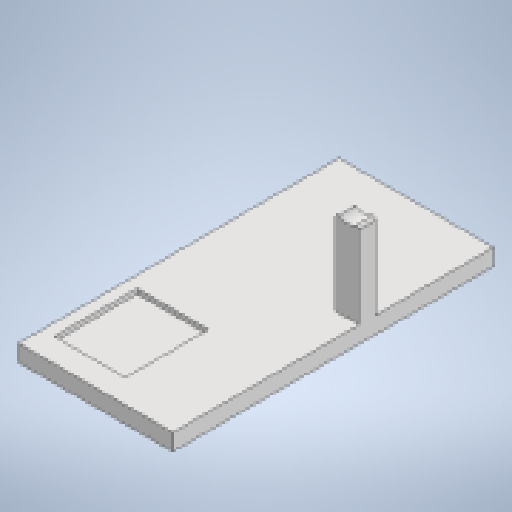
# Autodesk Inventor part: body-1
Saved by Autodesk Inventor 2025 (Build 290162000, 162)
## iProperties
Created: 2026-01-27
Part Number: body-1
Material: 一般
Document SubType Name: Modeling
Designer: mahhy
Density: 1 g/cm^3
Appearance: 既定
Author: mahhy
Autodesk Inventor part; units mm, degrees
ref_plane "YZ Plane" through (0, 0, 0) normal (1, 0, 0) x (0, 1, 0)
ref_plane "XZ Plane" through (0, 0, 0) normal (0, 1, 0) x (-1, 0, 0)
ref_plane "XY Plane" through (0, 0, 0) normal (0, 0, 1) x (1, 0, 0)
sketch "底面スケッチ" plane through (0, 0, 0) normal (0, 1, 0) x (-1, 0, 0)
  line L0 (0, 0) -> (65, 0)
  line L1 (65, 0) -> (65, -140)
  line L2 (65, -140) -> (0, -140)
  line L3 (0, -140) -> (0, 0)
  dimension "d0" = 65
  dimension "d1" = 140
  constraints: 8 end point, 2 parallel, 1 horizontal, 1 perpendicular
  measures "d0" distance of L1.end L2.end
  measures "d1" distance of L0.end L1.end
extrude "底面" add sketch "底面スケッチ" along normal blind 7
sketch "スケッチ2" plane through (0, 7, 0) normal (0, 1, 0) x (1, 0, 0)
  line L0 (-60, 10) -> (-30, 10)
  line L1 (-30, 10) -> (-30, 45)
  line L2 (-30, 45) -> (-60, 45)
  line L3 (-60, 45) -> (-60, 10)
  line L4 (-65, 0) -> (0, 0) projected
  line L5 (-65, 140) -> (-65, 0) projected
  dimension "d12" = 30
  dimension "d13" = 35
  dimension "d15" = 5
  constraints: 8 end point, 2 parallel, 1 horizontal, 1 perpendicular
  measures "d12" distance of L2.end L1.end
  measures "d13" distance of L1.end L0.end
  measures "d15" distance between parallel lines of L5 L3
extrude "溝" cut sketch "スケッチ2" against normal blind 2
sketch "スケッチ3" plane through (0, 7, 0) normal (0, 1, 0) x (1, 0, 0)
  line L0 (0, 0) -> (0, 140) projected
  line L1 (0, 85.5) -> (-10, 85.5)
  line L2 (-10, 85.5) -> (-10, 78.5)
  line L3 (-10, 78.5) -> (0, 78.5)
  line L4 (0, 78.5) -> (0, 85.5)
  line L5 (-65, 0) -> (0, 0) projected
  point P0 (0, 78.5)
  dimension "d18" = 10
  dimension "d19" = 7
  dimension "d20" = 78.5
  constraints: 8 end point, 2 parallel, 1 horizontal, 1 perpendicular, 1 point on line
  measures "d18" distance of L3.end L2.end
  measures "d19" distance of L2.end L1.end
  measures "d20" distance between parallel lines of L5 L3
extrude "押し出し3" add sketch "スケッチ3" along normal blind 41
sketch "スケッチ4" plane through (0, 7, -85.5) normal (0, 0, -1) x (-1, 0, 0)
  line L0 (0, 41) -> (10, 41) projected
  circle A0 centre (5, 41) radius 6.5
  line L1 (10, 0) -> (10, 41) projected
  point P0 (0, -7)
  point P1 (10.3848, 39)
  point P2 (-0.3848, 39)
  dimension "d25" = 13
  constraints: 1 centre point, 1 midpoint
  measures "d25" diameter of A0
extrude "押し出し4" cut sketch "スケッチ4" against normal blind 39
fillet "フィレット1" radius 1 2 edges at (-10, 43.8467, -82) (0, 43.8467, -82)
sketch "スケッチ5" plane through (0, 7, 0) normal (0, 1, 0) x (1, 0, 0)
  line L0 (-51, 90) -> (-10, 90)
  line L1 (-8, 92) -> (-8, 133)
  line L2 (-10, 135) -> (-51, 135)
  line L3 (-53, 133) -> (-53, 92)
  line L4 (0, 140) -> (-65, 140) projected
  line L5 (0, 85.5) -> (0, 140) projected
  arc A0 (-53, 92) -> (-51, 90) centre (-51, 92) ccw
  arc A1 (-51, 135) -> (-53, 133) centre (-51, 133) ccw
  arc A2 (-8, 133) -> (-10, 135) centre (-10, 133) ccw
  arc A3 (-10, 90) -> (-8, 92) centre (-10, 92) ccw
  point P0 (0, 0)
  point P1 (-53, 90)
  point P2 (-8, 135)
  point P3 (-8, 90)
  point P4 (-53, 135)
  dimension "d27" = 45
  dimension "d28" = 45
  dimension "d29" = 5
  dimension "d30" = 8
  dimension "d33" = 2
  constraints: 8 end point, 8 point on circle, 8 point on line, 8 tangent, 4 centre point, 3 equal radius, 2 parallel, 1 horizontal, 1 perpendicular
  measures "d27" distance of point (-53, 135) point (-8, 135)
  measures "d28" distance of point (-8, 90) point (-8, 135)
  measures "d29" distance between parallel lines of L4 L2
  measures "d30" distance between parallel lines of L5 L1
  measures "d33" radius of A0
extrude "ケース用溝" cut sketch "スケッチ5" against normal blind 3
equation "\"d28\" = d27"
